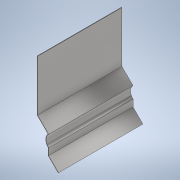
# Autodesk Inventor part: back
Saved by Autodesk Inventor 2020 (Build 240168000, 168)
## iProperties
Created: 2020-04-30
Part Number: back
Material: Generic
Document SubType Name: Modeling
Designer: LENOVO
Density: 1 g/cm^3
Appearance: Default
Author: LENOVO
Autodesk Inventor part; units mm, degrees
ref_plane "YZ Plane" through (0, 0, 0) normal (1, 0, 0) x (0, 1, 0)
ref_plane "XZ Plane" through (0, 0, 0) normal (0, 1, 0) x (-1, 0, 0)
ref_plane "XY Plane" through (0, 0, 0) normal (0, 0, 1) x (1, 0, 0)
sketch "Sketch1" plane through (0, 0, 0) normal (0, 0, 1) x (1, 0, 0)
  circle A0 centre (-0.0003, -247.8) radius 2.5
  line L0 (-100, -150) -> (-36.4384, -213.5616)
  line L1 (-100, -150) -> (-50, -150) construction
  line L2 (-36.4384, -213.5616) -> (-36.4394, -213.5606)
  line L3 (-35.3556, -283.1553) -> (-35.3556, -323.1553)
  line L4 (-35.3556, -283.1553) -> (4.6444, -283.1553) construction
  line L5 (-35.3556, -323.1553) -> (21.2129, -379.7239)
  arc A1 (-36.4384, -213.5616) -> (-35.3556, -283.1553) centre (-0.0003, -247.8) ccw
  line L6 (-32.3556, -281.8901) -> (-32.3556, -321.9127)
  line L7 (-32.3556, -321.9127) -> (25.4556, -379.7239)
  line L8 (-97, -148.7574) -> (-32.1971, -213.5602)
  arc A2 (-32.1971, -213.5602) -> (-32.3556, -281.8901) centre (-0.0003, -247.8) ccw
  line L9 (21.2129, -379.7239) -> (25.4556, -379.7239)
  line L10 (-100, -150) -> (-100, 150)
  line L11 (-97, -148.7574) -> (-97, 150)
  line L12 (-100, 150) -> (-97, 150)
  dimension "d0" = 5
  dimension "d1" = 45
  dimension "d3" = 50
  dimension "d5" = 40
  dimension "d6" = 90
  dimension "d7" = 80
  dimension "d8" = 135
  dimension "d13" = 3
  dimension "d16" = 3
  dimension "d17" = 3
  dimension "d19" = 35.3553
  dimension "d20" = 3
  dimension "d21" = 300
  constraints: 26 end point, 4 point on circle, 3 centre point, 3 parallel, 3 perpendicular, 2 coincident, 2 horizontal, 2 vertical, 1 collinear
  measures "d0" diameter of A0
  measures "d1" angle of L0 L1
  measures "d3" distance of A0.centre L4.start
  measures "d5" distance of L4.start L5.start
  measures "d6" angle of L3 L4
  measures "d7" distance of L5.start L9.start
  measures "d8" angle of L5 L3
  measures "d13" distance between parallel lines of L0 L8
  measures "d16" distance between parallel lines of L7 L5
  measures "d17" distance between parallel lines of L6 L3
  measures "d19" distance from line of L3 A1.centre
  measures "d20" distance between parallel lines of L10 L11
  measures "d21" distance of L1.start L10.end
extrude "Extrusion1" add sketch "Sketch1" against normal blind 494 contours L10 L12 L11 L8 A2 L6 L7 L9 L5 L3 A1 L0
body "Solid1"
